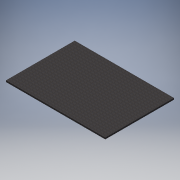
# Autodesk Inventor part: Grundriss
Saved by Autodesk Inventor 2017 (Build 210142000, 142)
## iProperties
Created: 2017-05-11
Part Number: Grundriss
Material: Beton
Document SubType Name: Modeling
Designer: Fake
Mass: 7.04139e+06 g
Surface Area: 607000 cm^2
Volume: 2.925e+06 cm^3
Density: 2.40731 g/cm^3
Appearance: Waschbeton - Grob
Author: Fake
Autodesk Inventor part; units mm, degrees
ref_plane "YZ Plane" through (0, 0, 0) normal (1, 0, 0) x (0, 1, 0)
ref_plane "XZ Plane" through (0, 0, 0) normal (0, 1, 0) x (-1, 0, 0)
ref_plane "XY Plane" through (0, 0, 0) normal (0, 0, 1) x (1, 0, 0)
sketch "Skizze1" plane through (0, 0, 0) normal (0, 0, 1) x (1, 0, 0)
  line L0 (-3250, 2250) -> (3250, 2250)
  line L1 (3250, 2250) -> (3250, -2250)
  line L2 (3250, -2250) -> (-3250, -2250)
  line L3 (-3250, -2250) -> (-3250, 2250)
  line L4 (-4550, 0) -> (4550, 0) projected
  line L5 (0, -3150) -> (0, 3150) projected
  point P0 (0, 0)
  dimension "d0" = 4500
  dimension "d1" = 6500
  constraints: 8 end point, 2 parallel, 1 horizontal, 1 perpendicular, 2 other
  measures "d0" distance of L2.end L0.start
  measures "d1" distance of L0.start L0.end
extrude "Extrusion1" add sketch "Skizze1" against normal blind 100
